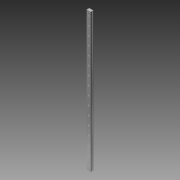
# Autodesk Inventor part: slide rail
Saved by Autodesk Inventor 2015 (Build 190159000, 159)
## iProperties
Created: 2015-01-29
Part Number: slide rail
Material: Generic
Document SubType Name: Modeling
Designer: Joseph
Density: 1 g/cm^3
Appearance: Chrome - Polished
Author: Joseph
Autodesk Inventor part; units mm, degrees
ref_plane "YZ Plane" through (0, 0, 0) normal (1, 0, 0) x (0, 1, 0)
ref_plane "XZ Plane" through (0, 0, 0) normal (0, 1, 0) x (-1, 0, 0)
ref_plane "XY Plane" through (0, 0, 0) normal (0, 0, 1) x (1, 0, 0)
sketch "Sketch1" plane through (0, 0, 0) normal (0, 0, 1) x (1, 0, 0)
  line L0 (6, 3.75) -> (-6, 3.75)
  line L1 (-6, -3.75) -> (6, -3.75)
  line L2 (6, 3.75) -> (-6, -3.75) construction
  line L3 (-6, 3.75) -> (6, -3.75) construction
  line L4 (-6, 0.25) -> (-4.75, 1.3065)
  line L5 (-4.75, 1.3065) -> (-6, 2.363)
  line L6 (-6, 3.75) -> (-6, 2.363)
  line L7 (-6, 0.25) -> (-6, -3.75)
  line L8 (6, 2.363) -> (4.75, 1.3065)
  line L9 (4.75, 1.3065) -> (6, 0.25)
  line L10 (6, -3.75) -> (6, 0.25)
  line L11 (6, 2.363) -> (6, 3.75)
  line L12 (-6, 0.25) -> (-6, 2.363) construction
  line L13 (6, 0.25) -> (6, 2.363) construction
  point P0 (0, 0)
  dimension "d0" = 12
  dimension "d1" = 7.5
  dimension "d2" = 9.5
  dimension "d3" = 1.387
  dimension "d4" = 4
  constraints: 28 end point, 8 parallel, 4 equal length, 2 midpoint, 2 perpendicular, 1 horizontal, 1 vertical
  measures "d0" distance of L1.end L1.start
  measures "d1" distance of L1.start L0.end
  measures "d2" distance of L8.end L4.end
  measures "d3" distance of L8.start L0.start
  measures "d4" distance of L1.end L9.end
extrude "Extrusion1" add sketch "Sketch1" along normal blind 400
sketch "Sketch2" plane through (-6, 3.75, 0) normal (0, 1, 0) x (1, 0, 0)
  line L0 (12, 0) -> (0, 0) projected
  line L1 (12, -400) -> (0, -400) projected
  line L2 (6, -408.5071) -> (6, 2.3747) construction
  point P0 (6, 0)
  point P1 (6, -388)
  point P2 (6, -363)
  point P3 (6, -338)
  point P4 (6, -313)
  point P5 (6, -288)
  point P6 (6, -263)
  point P7 (6, -238)
  point P8 (6, -213)
  point P9 (6, -188)
  point P10 (6, -163)
  point P11 (6, -138)
  point P12 (6, -113)
  point P13 (6, -88)
  point P14 (6, -63)
  point P15 (6, -38)
  point P16 (6, -13)
  dimension "d7" = 12
  dimension "d10" = 25
  constraints: 2 end point, 1 perpendicular, 1 point on line, 1 vertical, 15 other
  measures "d7" distance from line of L1 point (6, -388)
  measures "d10" distance of point (6, -388) point (6, -363)
hole "Hole1" at (0, 3.75, 388) at (0, 3.75, 363) at (0, 3.75, 338) at (0, 3.75, 313) at (0, 3.75, 288) at (0, 3.75, 263) at (0, 3.75, 238) at (0, 3.75, 213) at (0, 3.75, 188) at (0, 3.75, 163) at (0, 3.75, 138) at (0, 3.75, 113) at (0, 3.75, 88) at (0, 3.75, 63) at (0, 3.75, 38) at (0, 3.75, 13) direction (0, -1, 0) diameter 4 end through all counterbore diameter 6 counterbore depth 4.5
body "Solid1"
